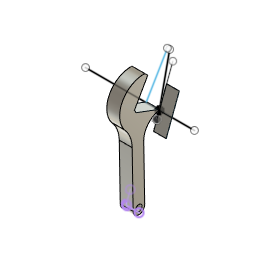
wrench 2 v5 (Autodesk Fusion 360 design; units mm, degrees)
Autodesk Fusion 360 part; units mm, degrees
note: some values were not read from the file. Chosen so that the rebuilt part matches the saved one: which face or edge a step refers to; a side. Set by a fixed rule: which sketch regions a step uses.
sketch "Sketch1" plane through (0, 0, 0) normal (1, 0, 0) x (0, 1, 0)
  circle A0 centre (0, 0) radius 5.3975
  circle A1 centre (0, 0) radius 9.9695
  line L0 (9.968, 0.174) -> (8.2973, 95.885)
  line L1 (-9.968, -0.174) -> (-11.6447, 95.885)
  line L2 (0, 2.5) -> (0, 20)
  line L3 (8.2973, 95.885) -> (-11.6447, 95.885)
  arc A2 (26.9075, 126.0089) -> (8.2973, 95.885) centre (41.0573, 96.4568) ccw
  arc A3 (35.56, 129.54) -> (26.9075, 126.0089) centre (61.0833, 54.6322) ccw
  line L4 (35.56, 129.54) -> (-5.08, 144.78)
  line L5 (-5.08, 144.78) -> (-7.62, 149.86)
  line L6 (-7.62, 149.86) -> (15.24, 190.5)
  line L7 (15.24, 190.5) -> (10.16, 195.58)
  arc A4 (10.16, 195.58) -> (-25.4, 129.54) centre (8.6053, 153.8233) ccw
  arc A5 (-11.6447, 95.885) -> (-25.4, 129.54) centre (-61.8377, 95.0089) ccw
  line L8 (15.24, 116.6313) -> (-25.4, 129.54)
  dimension "d1" = 10.795
  dimension "d2" = 19.939
  dimension "d3" = 1
  dimension "d4" = 1
  dimension "d5" = 95.885
  dimension "d6" = 19.942
  constraint coincident A0.centre A1.centre
  constraint concentric A0 A1
  constraint coincident A1 L0.start
  constraint tangent A1 L0
  constraint coincident A1 L1.start
  constraint tangent A1 L1
  constraint horizontal L0.end L1.end
  constraint tangent L0 A2
  constraint tangent A2 A3
  constraint tangent L1 A5
  constraint coincident A2 L8.start
  measures "d1" diameter of A0
  measures "d2" diameter of A1
  measures "d3" angle of L1 L2
  measures "d4" angle of L0 L2
  measures "d5" distance of A0.centre L3
  measures "d6" distance of L0.end L1.end
sketch "Sketch2" plane through (0, 0, 0) normal (1, 0, 0) x (0, 1, 0)
extrude "Extrude1" add sketch "Sketch1" along normal mid plane 22.225 makes body 1
sketch "Sketch3" plane through (0, 46.9726, 125.2603) normal (0, 0.351123, 0.936329) x (-1, 0, 0)
  line L0 (11.1125, 55.5922) -> (-11.1125, 55.5922)
  line L1 (-11.1125, 55.5922) -> (-11.1125, 12.1887)
  line L2 (-11.1125, 12.1887) -> (11.1125, 12.1887)
  line L3 (11.1125, 12.1887) -> (11.1125, 55.5922)
sketch "Sketch4" plane through (11.1125, 0, 0) normal (1, 0, 0) x (0, 1, 0)
  circle A0 centre (0, 0) radius 5.3975
  arc A1 (-9.968, -0.174) -> (9.968, 0.174) centre (0, 0) ccw
  line L0 (9.968, 0.174) -> (8.2973, 95.885)
  arc A2 (26.9075, 126.0089) -> (8.2973, 95.885) centre (41.0573, 96.4568) ccw
  arc A3 (35.56, 129.54) -> (26.9075, 126.0089) centre (61.0833, 54.6322) ccw
  line L1 (35.56, 129.54) -> (-5.08, 144.78)
  line L2 (-5.08, 144.78) -> (-7.62, 149.86)
  line L3 (-7.62, 149.86) -> (15.24, 190.5)
  line L4 (15.24, 190.5) -> (10.16, 195.58)
  arc A4 (10.16, 195.58) -> (-25.4, 129.54) centre (8.6053, 153.8233) ccw
  arc A5 (-11.6447, 95.885) -> (-25.4, 129.54) centre (-61.8377, 95.0089) ccw
  line L5 (-11.6447, 95.885) -> (-9.968, -0.174)
  line L6 (47.6205, 161.7013) -> (25.1594, 101.805)
  line L7 (-5.08, 144.78) -> (35.56, 129.54)
  constraint coincident A3.start L6
  constraint perpendicular L6 L7
extrude "Extrude2" add sketch "Sketch4" along normal blind 21.7678 thin wall 0.254 on the left separate body open curves L6 makes body 2
sketch "Sketch5" plane through (32.8803, 0, 0) normal (1, 0, 0) x (0, 1, 0)
  line L0 (25.3972, 101.7158) -> (47.8583, 161.6121)
  line L1 (47.8583, 161.6121) -> (47.6205, 161.7013)
  line L2 (47.6205, 161.7013) -> (25.1594, 101.805)
  line L3 (25.1594, 101.805) -> (25.3972, 101.7158)
sketch "Sketch6" plane through (32.8803, 0, 0) normal (1, 0, 0) x (0, 1, 0)
sketch "Sketch7" plane through (0, 0, 0) normal (0, 1, 0) x (1, 0, 0)
sketch "Sketch8" plane through (0, 46.9726, 125.2603) normal (0, 0.351123, 0.936329) x (1, 0, 0)
sketch "Sketch9" plane through (32.8803, 0, 0) normal (1, 0, 0) x (0, 1, 0)
sketch "Sketch10" plane through (0, 0, 0) normal (1, 0, 0) x (0, 1, 0)
sketch "Sketch11" plane through (0, 0, 0) normal (0, 0, 1) x (1, 0, 0)
sketch "Sketch12" plane through (0, 0, 0) normal (0, 0, 1) x (1, 0, 0)
sketch "Sketch13" plane through (0, 0, 0) normal (0, 1, 0) x (1, 0, 0)
sketch "Sketch14" plane through (32.8803, 0, 0) normal (1, 0, 0) x (0, 1, 0)
sketch "Sketch15" plane through (0, 0, 0) normal (0, 0, 1) x (1, 0, 0)
sketch "Sketch16" plane through (0, 0, 0) normal (0, 1, 0) x (1, 0, 0)
sketch "Sketch17" plane through (0, 0, 0) normal (1, 0, 0) x (0, 1, 0)
sketch "Sketch18" plane through (0, 0, 0) normal (1, 0, 0) x (0, 1, 0)
sketch "Sketch19" plane through (0, 0, 0) normal (0, 0, 1) x (1, 0, 0)
sketch "Sketch20" plane through (0, 0, 0) normal (1, 0, 0) x (0, 1, 0)
sketch "Sketch21" plane through (0, 0, 0) normal (0, 0, 1) x (1, 0, 0)
sketch "Sketch22" plane through (0, 0, 0) normal (0, 1, 0) x (1, 0, 0)
sketch "Sketch23" plane through (32.8803, 0, 0) normal (1, 0, 0) x (0, 1, 0)
sketch "Sketch24" plane through (32.8803, 0, 0) normal (1, 0, 0) x (0, 1, 0)
sketch "Sketch25" plane through (0, -11.1748, 4.1905) normal (0, 0.936329, -0.351123) x (-1, 0, 0)
  line L0 (-11.1125, 104.1571) -> (-11.1125, 168.1263)
  line L1 (-11.1125, 168.1263) -> (-32.8803, 168.1263)
  line L2 (-32.8803, 168.1263) -> (-32.8803, 104.1571)
  line L3 (-32.8803, 104.1571) -> (-11.1125, 104.1571)
  line L4 (-11.1125, 198.3034) -> (-11.1125, 120.2743)
  line L5 (-71.4242, 132.461) -> (116.1687, 132.461)
  line L6 (-1.75, 0) -> (-22.5, 0)
  line L7 (-1.6144, 209.8168) -> (-11.1125, 132.461)
  line L8 (2.3104, 209.77) -> (11.8027, 132.461)
  line L9 (0, 1.6386) -> (0, 21.0674)
  dimension "d12" = 132.461
  dimension "d13" = 7
  dimension "d14" = 7
  constraint vertical L4
  constraint perpendicular L4 L5
  constraint coincident L0 L4.end
  constraint coincident L0 L7.end
  constraint coincident L5 L7.end
  constraint coincident L5 L8.end
  measures "d12" distance of L5 L6
  measures "d13" angle of L8 L9
  measures "d14" angle of L7 L9
sketch "Sketch26" plane through (0, -11.1748, 4.1905) normal (0, 0.936329, -0.351123) x (-1, 0, 0)
